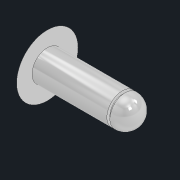
# Autodesk Inventor part: M5 x 12.7 Rivet
Saved by Autodesk Inventor 2022 (Build 260153000, 153)
## iProperties
Created: 2022-09-23
Part Number: M5 x 12.7 Rivet
Material: Generic
Document SubType Name: Modeling
Designer: robpl
Density: 1 g/cm^3
Appearance: Aluminum - Dark
Author: robpl
Autodesk Inventor part; units mm, degrees
ref_plane "YZ Plane" through (0, 0, 0) normal (1, 0, 0) x (0, 1, 0)
ref_plane "XZ Plane" through (0, 0, 0) normal (0, 1, 0) x (-1, 0, 0)
ref_plane "XY Plane" through (0, 0, 0) normal (0, 0, 1) x (1, 0, 0)
sketch "Sketch1" plane through (0, 0, 0) normal (0, 0, 1) x (1, 0, 0)
  line L0 (0, 0) -> (0, 5)
  line L1 (0, 0) -> (12.7, 0)
  line L2 (12.7, 0) -> (12.7, 2.5)
  line L3 (12.7, 2.5) -> (0, 2.5)
  line L4 (0, 2.5) -> (0, 0)
  circle A0 centre (8.6603, 0) radius 10
  line L5 (-11, 1) -> (-1, 1)
  line L6 (-1, 1) -> (-1, -1)
  line L7 (-1, -1) -> (-11, -1)
  line L8 (-11, -1) -> (-11, 1)
  line L9 (0, 0) -> (-1, 0)
  line L10 (12.7, 2.5) -> (12.2, 2.5)
  line L11 (12.2, 2.5) -> (12.2, 2)
  line L12 (12.2, 2) -> (12.7, 2)
  line L13 (12.7, 2) -> (12.7, 2.5)
  circle A1 centre (12.7, 0) radius 2.5
  line L14 (12.7, 0) -> (15.2, 0)
  point P0 (-1.2896, 1)
  dimension "d3" = 20
  dimension "d0" = 5
  dimension "d1" = 12.7
  dimension "d2" = 2.5
  dimension "d4" = 1
  dimension "d5" = 1
  dimension "d6" = 1
  dimension "d7" = 10
  dimension "d8" = 0.5
  dimension "d9" = 0.5
  constraints: 30 end point, 6 parallel, 4 horizontal, 3 perpendicular, 2 point on circle, 1 centre point, 1 coincident, 1 midpoint, 1 point on line, 1 vertical, 3 other
  measures "d0" distance of L0.start L0.end
  measures "d1" distance of L3.end L2.end
  measures "d2" distance of L2.end L1.end
  measures "d4" distance between parallel lines of L5 L1
  measures "d5" distance between parallel lines of L0 L6
  measures "d6" distance between parallel lines of L1 L7
  measures "d7" distance of L5.start L5.end
  measures "d8" distance of L12.end L11.end
  measures "d9" distance of L11.end L10.end
revolve "Revolution1" add sketch "Sketch1" angle 360 about axis through (0, 0, 0) along (1, 0, 0) contours L9 L6 L5 A0 L0 | L0 L3 L11 A1 L1 | A1 L11 L12 L2 L1 | L2 A1 L14
equation "\"d6\" = d4"
body "Solid1"
